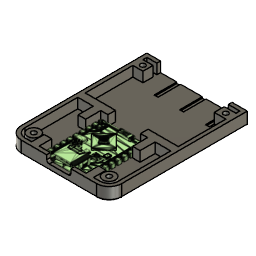
PS1MemCard (Autodesk Fusion 360 design; units mm, degrees)
Autodesk Fusion 360 part; units mm, degrees
sketch "Sketch1" plane through (0, 0, 0) normal (0, 0, 1) x (1, 0, 0)
  line L0 (-7.8737, 2.48) -> (28.1263, 2.48)
  line L1 (28.1263, 2.48) -> (28.1263, -15.52)
  line L2 (28.1263, -15.52) -> (-7.8737, -15.52)
  line L3 (-7.8737, -15.52) -> (-7.8737, 2.48)
  dimension "d1" = 36
  dimension "d2" = 18
  constraint horizontal L0
  constraint vertical L1
  constraint horizontal L2
  constraint vertical L3
  measures "d1" distance of L0.start L0.end
  measures "d2" distance of L0.start L2.end
other "Base Mesh Feature2"
sketch "Sketch2" plane through (0, 0, 0) normal (0, 0, 1) x (1, 0, 0)
  line L0 (-20, 0) -> (-20, -50)
  line L1 (20, 0) -> (20, -50)
  line L2 (-15, -55) -> (15, -55)
  line L3 (-20, 0) -> (20, 0)
  arc A0 (-20, -50) -> (-15, -55) centre (-15, -50) ccw
  arc A1 (15, -55) -> (20, -50) centre (15, -50) ccw
  line L4 (20, 0) -> (18.5, 0)
  line L5 (-20, 0) -> (-18.5, 0)
  line L6 (18.5, 0) -> (-18.5, 0)
  line L7 (-18.5, 0) -> (-18.5, -50)
  line L8 (-15, -53.5) -> (15, -53.5)
  line L9 (18.5, -50) -> (18.5, 0)
  arc A2 (15, -53.5) -> (18.5, -50) centre (15, -50) ccw
  arc A3 (-18.5, -50) -> (-15, -53.5) centre (-15, -50) ccw
  line L10 (18.5, 0) -> (13.5, 0)
  line L11 (18.5, -1.5) -> (18.5, 0)
  line L12 (-18.5, 0) -> (-15, 0)
  line L13 (-15, -1.5) -> (-18.5, -1.5)
  line L14 (-18.5, -1.5) -> (-18.5, 0)
  line L15 (3.5957, 0) -> (2.0957, 0)
  line L16 (2.0957, 0) -> (2.0957, -7)
  line L17 (3.5957, -7) -> (3.5957, 0)
  line L18 (-6.5571, 0) -> (-8.0571, 0)
  line L19 (-8.0571, 0) -> (-8.0571, -7)
  line L20 (-6.5571, -7) -> (-6.5571, 0)
  line L21 (18.5, 0) -> (18.5, -26)
  line L22 (-18.5, 0) -> (-18.5, -26)
  line L23 (18.5, -29) -> (18.5, -26)
  line L24 (-18.5, -29) -> (-18.5, -26)
  line L25 (9.2963, -53.5) -> (12.2963, -53.5)
  line L26 (12.2963, -53.5) -> (12.2963, -48.5)
  line L27 (12.2963, -48.5) -> (9.2963, -48.5)
  line L28 (9.2963, -48.5) -> (9.2963, -53.5)
  line L29 (-9.3535, -53.5) -> (-12.3535, -53.5)
  line L30 (-12.3535, -53.5) -> (-12.3535, -48.5)
  line L31 (-12.3535, -48.5) -> (-9.3535, -48.5)
  line L32 (-9.3535, -48.5) -> (-9.3535, -53.5)
  line L33 (-18.5, -7.0506) -> (-14.5, -7.0506)
  line L34 (-14.5, -7.0506) -> (-14.5, -3.0506)
  line L35 (-14.5, -3.0506) -> (-18.5, -3.0506)
  line L36 (-18.5, -3.0506) -> (-18.5, -7.0506)
  line L37 (18.5, -7.0468) -> (14.5, -7.0468)
  line L38 (13.8751, -3.0468) -> (18.5, -3.0468)
  line L39 (18.5, -3.0468) -> (18.5, -7.0468)
  line L40 (18.5, -29) -> (6.5, -29)
  line L41 (6.5, -29) -> (6.5, -26)
  line L42 (6.5, -26) -> (18.5, -26)
  line L43 (18.5, -26) -> (18.5, -29)
  line L44 (-18.5, -29) -> (-6.5, -29)
  line L45 (-6.5, -29) -> (-6.5, -26)
  line L46 (-6.5, -26) -> (-18.5, -26)
  line L47 (-18.5, -26) -> (-18.5, -29)
  line L48 (-9.3535, -48.5) -> (-9.3535, -29)
  line L49 (9.2963, -48.5) -> (9.2963, -29)
  line L50 (-9.3535, -29) -> (-12.3535, -29)
  line L51 (-12.3535, -29) -> (-12.3535, -35)
  line L52 (-12.3535, -35) -> (-9.3535, -35)
  line L53 (-9.3535, -35) -> (-9.3535, -29)
  line L54 (9.2963, -29) -> (12.2963, -29)
  line L55 (12.2963, -29) -> (12.2963, -35)
  line L56 (12.2963, -35) -> (9.2963, -35)
  line L57 (9.2963, -35) -> (9.2963, -29)
  circle A4 centre (-15, -50) radius 2.5
  circle A5 centre (15, -50) radius 2.5
  line L58 (12.3751, 0) -> (13.8751, 0)
  line L59 (13.8751, 0) -> (13.8751, -7)
  line L60 (12.3751, -7) -> (12.3751, 0)
  line L61 (18.5, -1.5) -> (13.8751, -1.5)
  line L62 (-18.5, -1.5) -> (-14.5, -1.5)
  line L63 (-14.5, -1.5) -> (-14.5, 0)
  line L64 (-14.5, 0) -> (-18.5, 0)
  line L65 (-18.5, 0) -> (-18.5, -1.5)
  line L66 (-6.5571, -7) -> (-6.5571, -9)
  line L67 (-6.5571, -9) -> (-8.0571, -9)
  line L68 (-8.0571, -9) -> (-8.0571, -7)
  line L69 (3.5957, -7) -> (3.5957, -9)
  line L70 (3.5957, -9) -> (2.0957, -9)
  line L71 (2.0957, -9) -> (2.0957, -7)
  line L72 (13.8751, -7) -> (13.8751, -9)
  line L73 (13.8751, -9) -> (12.3751, -9)
  line L74 (12.3751, -9) -> (12.3751, -7)
  line L75 (14.5, -7.0468) -> (13.8751, -7.0468)
  line L76 (13.8751, -7.0468) -> (13.8751, -3.0468)
  point P0 (18.5, -53.5)
  dimension "d9" = 5
  dimension "d10" = 5
  dimension "d20" = 1.5
  dimension "d21" = 1.5
  dimension "d22" = 37
  dimension "d23" = 53.5
  dimension "d24" = 3.5
  dimension "d25" = 3.5
  dimension "d28" = 5
  dimension "d29" = 1.5
  dimension "d30" = 3.5
  dimension "d31" = 1.5
  dimension "d32" = 1.5
  dimension "d33" = 7
  dimension "d34" = 1.5
  dimension "d35" = 7
  dimension "d37" = 26
  dimension "d39" = 3
  dimension "d41" = 3
  dimension "d42" = 3
  dimension "d43" = 5
  dimension "d44" = 3
  dimension "d45" = 5
  dimension "d53" = 4
  dimension "d54" = 4
  dimension "d55" = 4
  dimension "d56" = 4
  dimension "d57" = 12
  dimension "d58" = 3
  dimension "d59" = 12
  dimension "d60" = 3
  dimension "d61" = 3
  dimension "d62" = 6
  dimension "d63" = 3
  dimension "d64" = 6
  dimension "d65" = 5
  dimension "d66" = 5
  dimension "d79" = 1.5
  dimension "d80" = 7
  dimension "d83" = 4
  dimension "d84" = 1.5
  dimension "d85" = 2
  dimension "d86" = 1.5
  dimension "d87" = 2
  dimension "d88" = 1.5
  dimension "d89" = 2
  constraint perpendicular L1 L3
  constraint tangent L0 A0
  constraint tangent L2 A0
  constraint tangent L1 A1
  constraint tangent L2 A1
  constraint perpendicular L1 L4
  constraint horizontal L5
  constraint perpendicular L0 L5
  constraint horizontal L6
  constraint vertical L7
  constraint horizontal L8
  constraint vertical L9
  constraint coincident P0 L9
  constraint coincident P0 L8
  constraint tangent L9 A2
  constraint tangent L8 A2
  constraint tangent L7 A3
  constraint tangent L8 A3
  constraint horizontal L10
  constraint vertical L11
  constraint horizontal L12
  constraint horizontal L13
  constraint vertical L14
  constraint horizontal L15
  constraint vertical L16
  constraint vertical L17
  constraint coincident L3 L15.start
  constraint coincident L6 L15.start
  constraint horizontal L18
  constraint vertical L19
  constraint vertical L20
  constraint coincident L3 L18.start
  constraint coincident L6 L18.start
  constraint perpendicular L12 L22
  constraint vertical L23
  constraint vertical L24
  constraint horizontal L25
  constraint vertical L26
  constraint horizontal L27
  constraint vertical L28
  constraint coincident L8 L25.start
  constraint horizontal L29
  constraint vertical L30
  constraint horizontal L31
  constraint vertical L32
  constraint coincident L8 L29.start
  constraint horizontal L33
  constraint vertical L34
  constraint horizontal L35
  constraint vertical L36
  constraint coincident L7 L33.start
  constraint horizontal L37
  constraint horizontal L38
  constraint vertical L39
  constraint coincident L21 L37.start
  constraint horizontal L40
  constraint vertical L41
  constraint horizontal L42
  constraint vertical L43
  constraint horizontal L44
  constraint vertical L45
  constraint horizontal L46
  constraint vertical L47
  constraint coincident L44 L48.end
  constraint perpendicular L44 L48
  constraint coincident L40 L49.end
  constraint perpendicular L40 L49
  constraint horizontal L50
  constraint vertical L51
  constraint horizontal L52
  constraint vertical L53
  constraint horizontal L54
  constraint vertical L55
  constraint horizontal L56
  constraint vertical L57
  constraint concentric A3 A4
  constraint concentric A1 A5
  constraint horizontal L58
  constraint vertical L59
  constraint vertical L60
  constraint coincident L3 L58.start
  constraint coincident L6 L58.start
  constraint coincident L59 L61.end
  constraint horizontal L62
  constraint vertical L63
  constraint horizontal L64
  constraint vertical L65
  constraint vertical L66
  constraint horizontal L67
  constraint vertical L68
  constraint vertical L69
  constraint horizontal L70
  constraint vertical L71
  constraint vertical L72
  constraint horizontal L73
  constraint vertical L74
  constraint horizontal L75
  constraint vertical L76
  constraint coincident L59 L38.start
  measures "d9" radius of A0
  measures "d10" radius of A1
  measures "d20" distance of L1.start L4.end
  measures "d21" distance of L0.start L5.end
  measures "d22" distance of L4.end L5.end
  measures "d23" distance of L4.end P0
  measures "d24" radius of A2
  measures "d25" radius of A3
  measures "d28" distance of L4.end L10.end
  measures "d29" distance of L4.end L11.start
  measures "d30" distance of L5.end L12.end
  measures "d31" distance of L5.end L13.end
  measures "d32" distance of L15.start L15.end
  measures "d33" distance of L15.start L17.start
  measures "d34" distance of L18.start L18.end
  measures "d35" distance of L18.start L20.start
  measures "d37" distance of L5.end L22.end
  measures "d39" distance of L21.end L23.start
  measures "d41" distance of L22.end L24.start
  measures "d42" distance of L25.start L25.end
  measures "d43" distance of L25.start L27.end
  measures "d44" distance of L29.start L29.end
  measures "d45" distance of L29.start L31.end
  measures "d53" distance of L33.start L33.end
  measures "d54" distance of L33.start L35.end
  measures "d55" distance of L37.start L37.end
  measures "d56" distance of L37.start L38.end
  measures "d57" distance of L23.start L40.end
  measures "d58" distance of L23.start L21.end
  measures "d59" distance of L24.start L44.end
  measures "d60" distance of L24.start L22.end
  measures "d61" distance of L48.end L50.end
  measures "d62" distance of L48.end L52.end
  measures "d63" distance of L49.end L54.end
  measures "d64" distance of L49.end L56.end
  measures "d65" diameter of A4
  measures "d66" diameter of A5
  measures "d79" distance of L58.start L58.end
  measures "d80" distance of L58.start L60.start
  measures "d83" distance of L13.end L62.end
  measures "d84" distance of L19.end L20.start
  measures "d85" distance of L19.end L67.end
  measures "d86" distance of L16.end L17.start
  measures "d87" distance of L16.end L70.end
  measures "d88" distance of L60.start L59.end
  measures "d89" distance of L60.start L73.end
other "Modify1"
extrude "Extrude1" add sketch "Sketch2" against normal blind 1 contours L0 L1 L2 L3 A0 A1 L4 L5 L7 L8 L9 A2 A3 L11 L14 L21 L22 L23 L24 L25 L29 L36 L39 L43 L47 L65 | L3 L6 L7 L12 L13 L14 L22 L62 L63 L64 L65 | L3 L6 L7 L8 L9 L13 L16 L17 L19 L20 L21 L22 L28 L32 L33 L34 L35 L37 L40 L41 L42 L44 L45 L46 L48 L49 L53 L57 L60 L62 L63 L66 L67 L68 L69 L70 L71 L72 L73 L74 L75 | L7 L22 L33 L34 L35 L36 | L3 L6 L18 L19 L20 L66 L67 L68 | L7 L24 L44 L45 L46 L47 L50 | L3 L6 L9 L10 L11 L21 L59 L61 | L3 L6 L15 L16 L17 L69 L70 L71 | L7 L8 A3 L30 L31 L44 L48 L51 L52 | L3 L6 L10 L58 L59 L60 L72 L73 L74 L76 | L9 L21 L38 L59 L61 | L44 L48 L50 L51 L52 L53 | L9 L21 L37 L38 L39 L59 L72 L75 L76 | L8 L29 L30 L31 L32 | L9 L23 L40 L41 L42 L43 L54 | L8 L9 A2 L26 L27 L40 L49 L55 L56 | L8 L25 L26 L27 L28 | L40 L49 L54 L55 L56 L57 | A4 | A5 makes body 1
extrude "Extrude4" add sketch "Sketch2" along normal blind 4 contours L0 L1 L2 L3 A0 A1 L4 L5 L7 L8 L9 A2 A3 L11 L14 L21 L22 L23 L24 L25 L29 L36 L39 L43 L47 L65 | L3 L6 L7 L12 L13 L14 L22 L62 L63 L64 L65 | L7 L22 L33 L34 L35 L36 | L7 L24 L44 L45 L46 L47 L50 | L3 L6 L9 L10 L11 L21 L59 L61 | L44 L48 L50 L51 L52 L53 | L9 L21 L37 L38 L39 L59 L72 L75 L76 | L8 L29 L30 L31 L32 | L9 L23 L40 L41 L42 L43 L54 | L8 L25 L26 L27 L28 | L40 L49 L54 L55 L56 L57 | A4 | A5 bodies 1
sketch "Sketch4" plane through (0, 0, 0) normal (0, 1, 0) x (1, 0, 0)
  line L0 (-3.8349, -5.0627) -> (3.7734, -5.0627)
  line L1 (4.7734, -4.0627) -> (4.7734, -2.3553)
  line L2 (3.7734, -1.3553) -> (-3.8349, -1.3553)
  line L3 (-4.8349, -2.3553) -> (-4.8349, -4.0627)
  arc A0 (-3.8349, -1.3553) -> (-4.8349, -2.3553) centre (-3.8349, -2.3553) ccw
  arc A1 (4.7734, -2.3553) -> (3.7734, -1.3553) centre (3.7734, -2.3553) ccw
  arc A2 (3.7734, -5.0627) -> (4.7734, -4.0627) centre (3.7734, -4.0627) ccw
  arc A3 (-4.8349, -4.0627) -> (-3.8349, -5.0627) centre (-3.8349, -4.0627) ccw
  dimension "d48" = 1
  constraint horizontal L0
  constraint vertical L1
  constraint horizontal L2
  constraint vertical L3
  constraint tangent L2 A0
  constraint tangent L3 A0
  constraint tangent L1 A1
  constraint tangent L2 A1
  constraint equal A0 A1
  constraint tangent L0 A2
  constraint tangent L1 A2
  constraint equal A0 A2
  constraint tangent L0 A3
  constraint tangent L3 A3
  constraint equal A0 A3
  measures "d48" radius of A0
extrude "Extrude7" add sketch "Sketch2" along normal blind 2 separate body contours L0 L1 L2 L3 A0 A1 L4 L5 L7 L8 L9 A2 A3 L11 L14 L21 L22 L23 L24 L25 L29 L36 L39 L43 L47 L65 | L3 L6 L7 L12 L13 L14 L22 L62 L63 L64 L65 | L3 L6 L7 L8 L9 L13 L16 L17 L19 L20 L21 L22 L28 L32 L33 L34 L35 L37 L40 L41 L42 L44 L45 L46 L48 L49 L53 L57 L60 L62 L63 L66 L67 L68 L69 L70 L71 L72 L73 L74 L75 | L7 L22 L33 L34 L35 L36 | L3 L6 L18 L19 L20 L66 L67 L68 | L7 L24 L44 L45 L46 L47 L50 | L3 L6 L9 L10 L11 L21 L59 L61 | L3 L6 L15 L16 L17 L69 L70 L71 | L7 L8 A3 L30 L31 L44 L48 L51 L52 | L3 L6 L10 L58 L59 L60 L72 L73 L74 L76 | L9 L21 L38 L59 L61 | L44 L48 L50 L51 L52 L53 | L9 L21 L37 L38 L39 L59 L72 L75 L76 | L8 L29 L30 L31 L32 | L9 L23 L40 L41 L42 L43 L54 | L8 L9 A2 L26 L27 L40 L49 L55 L56 | L8 L25 L26 L27 L28 | L40 L49 L54 L55 L56 L57 | A4 | A5 makes body 2
move_body "Move1" bodies 2 to x (1, 0, 0) y (0, 1, 0) z (0, 0, 1) at (0, 0, 4)
ref_plane "WorkPlane1" through (-0.0307, -55, 3.209) normal (0, 1, 0) x (1, 0, 0)
extrude "Extrude5" cut sketch "Sketch4" along normal blind 10 from surface at -55 bodies 1 2
extrude "Extrude6" cut sketch "Sketch2" against normal blind 0.5 contours L3 L6 L18 L19 L20 L66 L67 L68 | L3 L6 L15 L16 L17 L69 L70 L71 | L3 L6 L10 L58 L59 L60 L72 L73 L74 L76 bodies 1
hole "Hole1" at (-15, -50, 6) direction (0, 0, -1) diameter 2 depth 5 tip angle 180 countersink diameter 5 countersink angle 90 bodies 1 2
hole "Hole2" at (15, -50, 6) direction (0, 0, -1) diameter 2 depth 5 tip angle 180 countersink diameter 5 countersink angle 90 bodies 1 2
hole "Hole3" at (-16.5881, -5.0215, 6) direction (0, 0, -1) diameter 2 depth 5 tip angle 180 countersink diameter 5 countersink angle 90 bodies 1 2
hole "Hole4" at (16.4664, -5.0546, 6) direction (0, 0, -1) diameter 2 depth 5 tip angle 180 countersink diameter 5 countersink angle 90 bodies 1 2
fillet "Fillet1" radius 0.5 5 edges at (-20, -25, 6) (-18.5355, -53.5355, 6) (0, -55, 6) (18.5355, -53.5355, 6) (20, -25, 6) on bodies 2
fillet "Fillet2" radius 0.5 5 edges at (20, -25, -1) (18.5355, -53.5355, -1) (0, -55, -1) (-18.5355, -53.5355, -1) (-20, -25, -1) on bodies 1
sketch "Sketch5" plane through (0, 0, 4) normal (0, 0, -1) x (1, 0, 0)
  circle A0 centre (16.4664, 5.0546) radius 1
  circle A1 centre (-16.5881, 5.0215) radius 1
  circle A2 centre (15, 50) radius 1
  circle A3 centre (-15, 50) radius 1
  line L0 (-4.8349, 45) -> (-4.8349, 55)
  line L1 (-4.8349, 55) -> (-15, 55)
  arc A4 (-15, 55) -> (-20, 50) centre (-15, 50) ccw
  line L2 (-20, 50) -> (-20, 0)
  line L3 (-20, 0) -> (20, 0)
  line L4 (20, 0) -> (20, 50)
  arc A5 (20, 50) -> (15, 55) centre (15, 50) ccw
  line L5 (15, 55) -> (4.7734, 55)
  line L6 (4.7734, 55) -> (4.7734, 45)
  line L7 (4.7734, 45) -> (-4.8349, 45)
  circle A6 centre (0.171, 37.3473) radius 2.5
  circle A7 centre (14.976, 22.0787) radius 1.5
  circle A8 centre (-14.8658, 22.0124) radius 1.5
  circle A9 centre (-14.8658, 13.9862) radius 1.5
  circle A10 centre (14.976, 13.9472) radius 1.5
  dimension "d104" = 5
  dimension "d107" = 3
  dimension "d108" = 3
  dimension "d135" = 3
  dimension "d136" = 3
  measures "d104" diameter of A6
  measures "d107" diameter of A7
  measures "d108" diameter of A8
  measures "d135" diameter of A9
  measures "d136" diameter of A10
sketch "Sketch6" plane through (0, 0, 0) normal (0, 0, 1) x (1, 0, 0)
  line L0 (-11.9858, 0.5093) -> (-9.9858, 0.5093)
  line L1 (-9.9858, 0.5093) -> (-9.9858, -9.4907)
  line L2 (-9.9858, -9.4907) -> (-11.9858, -9.4907)
  line L3 (-11.9858, -9.4907) -> (-11.9858, 0.5093)
  line L4 (-2.5141, 0.5093) -> (-0.5141, 0.5093)
  line L5 (-0.5141, 0.5093) -> (-0.5141, -9.4907)
  line L6 (-0.5141, -9.4907) -> (-2.5141, -9.4907)
  line L7 (-2.5141, -9.4907) -> (-2.5141, 0.5093)
  line L8 (7.4928, 0.5093) -> (9.4928, 0.5093)
  line L9 (9.4928, 0.5093) -> (9.4928, -9.4907)
  line L10 (9.4928, -9.4907) -> (7.4928, -9.4907)
  line L11 (7.4928, -9.4907) -> (7.4928, 0.5093)
  dimension "d118" = 2
  dimension "d119" = 10
  dimension "d120" = 2
  dimension "d121" = 10
  dimension "d122" = 2
  dimension "d123" = 10
  constraint horizontal L0
  constraint vertical L1
  constraint horizontal L2
  constraint vertical L3
  constraint horizontal L4
  constraint vertical L5
  constraint horizontal L6
  constraint vertical L7
  constraint horizontal L8
  constraint vertical L9
  constraint horizontal L10
  constraint vertical L11
  measures "d118" distance of L0.start L0.end
  measures "d119" distance of L0.start L2.end
  measures "d120" distance of L4.start L4.end
  measures "d121" distance of L4.start L6.end
  measures "d122" distance of L8.start L8.end
  measures "d123" distance of L8.start L10.end
extrude "Extrude10" cut sketch "Sketch6" along normal blind 5.5 bodies 2
extrude "Extrude11" cut sketch "Sketch2" along normal up to surface (5 mm away) contours L3 L6 L7 L8 L9 L13 L16 L17 L19 L20 L21 L22 L28 L32 L33 L34 L35 L37 L40 L41 L42 L44 L45 L46 L48 L49 L53 L57 L60 L62 L63 L66 L67 L68 L69 L70 L71 L72 L73 L74 L75 | L3 L6 L18 L19 L20 L66 L67 L68 | L3 L6 L15 L16 L17 L69 L70 L71 | L7 L8 A3 L30 L31 L44 L48 L51 L52 | L3 L6 L10 L58 L59 L60 L72 L73 L74 L76 | L9 L21 L38 L59 L61 | L8 L29 L30 L31 L32 | L8 L9 A2 L26 L27 L40 L49 L55 L56 | L8 L25 L26 L27 L28 bodies 2
extrude "Extrude8" add sketch "Sketch5" along normal blind 2.5 from surface at -1 separate body contours A6 makes body 3
extrude "Extrude9" add sketch "Sketch5" along normal blind 3.5 from surface at -1 separate body contours A7 | A8 | A9 | A10 makes body 4 at (-16.3584, -21.8631, 2.6667) makes body 5 at (13.4834, -21.9293, 2.6667) makes body 6 at (16.4685, -13.7979, 2.6667) makes body 7 at (-13.3733, -13.8368, 2.6667)
sketch "Sketch7" plane through (0, 0, 0) normal (0, 0, 1) x (1, 0, 0)
  line L0 (-7.1411, -0.0167) -> (-5.9972, -0.0167)
  line L1 (-5.9972, -0.0167) -> (-5.9972, -7.5452)
  line L2 (-6.4372, -7.9852) -> (-6.7011, -7.9852)
  line L3 (-7.1411, -7.5452) -> (-7.1411, -0.0167)
  line L4 (3.2039, -0.0167) -> (4.2098, -0.0167)
  line L5 (4.2098, -0.0167) -> (4.2098, -7.6552)
  line L6 (3.8798, -7.9852) -> (3.6439, -7.9852)
  line L7 (3.2039, -7.5452) -> (3.2039, -0.0167)
  arc A0 (-7.1411, -7.5452) -> (-6.7011, -7.9852) centre (-6.7011, -7.5452) ccw
  arc A1 (-6.4372, -7.9852) -> (-5.9972, -7.5452) centre (-6.4372, -7.5452) ccw
  arc A2 (3.2039, -7.5452) -> (3.6439, -7.9852) centre (3.6439, -7.5452) ccw
  arc A3 (3.8798, -7.9852) -> (4.2098, -7.6552) centre (3.8798, -7.6552) ccw
  dimension "d130" = 0.44
  dimension "d131" = 0.33
  constraint horizontal L0
  constraint vertical L1
  constraint horizontal L2
  constraint vertical L3
  constraint horizontal L4
  constraint vertical L5
  constraint horizontal L6
  constraint vertical L7
  constraint tangent L2 A0
  constraint tangent L3 A0
  constraint tangent L1 A1
  constraint tangent L2 A1
  constraint equal A0 A1
  constraint tangent L6 A2
  constraint tangent L7 A2
  constraint equal A0 A2
  constraint tangent L5 A3
  constraint tangent L6 A3
  measures "d130" radius of A0
  measures "d131" radius of A3
extrude "Extrude12" add sketch "Sketch7" along normal blind 3 from surface at 2 bodies 2
hidden bodies 2 3 5 6 4 7
